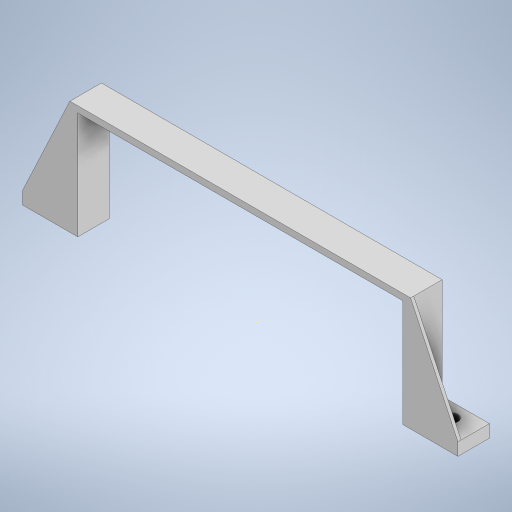
# Autodesk Inventor part: KVMMount
Saved by Autodesk Inventor 2023 (Build 270158000, 158)
## iProperties
Created: 2023-03-26
Part Number: KVMMount
Material: Generic
Document SubType Name: Modeling
Designer: lidang
Density: 1 g/cm^3
Appearance: Default
Author: lidang
Autodesk Inventor part; units mm, degrees
ref_plane "YZ Plane" through (0, 0, 0) normal (1, 0, 0) x (0, 1, 0)
ref_plane "XZ Plane" through (0, 0, 0) normal (0, 1, 0) x (-1, 0, 0)
ref_plane "XY Plane" through (0, 0, 0) normal (0, 0, 1) x (1, 0, 0)
sketch "Sketch1" plane through (0, 0, 0) normal (0, 0, 1) x (1, 0, 0)
  point P0 (0, 0)
sketch "Sketch2" plane through (0, 0, 0) normal (0, 0, 1) x (1, 0, 0)
  line L0 (-69, 0) -> (-69, 4)
  line L1 (-69, 4) -> (-54, 4)
  line L2 (-54, 4) -> (-54, 36)
  line L3 (-54, 36) -> (0, 36)
  line L4 (0, 36) -> (0, 34)
  line L5 (0, 34) -> (-51.5, 34)
  line L6 (-51.5, 34) -> (-51.5, 0)
  line L7 (-51.5, 0) -> (-69, 0)
  point P0 (0, 0)
  point P1 (-25.75, 34)
  point P2 (0, 35)
  dimension "d0" = 2
  dimension "d1" = 2.5
  dimension "d2" = 4
  dimension "d3" = 4
  dimension "d4" = 15
  dimension "d6" = 0
  dimension "d8" = 51.5
  dimension "d11" = 34
  constraints: 16 end point, 7 perpendicular, 2 midpoint, 1 vertical
  measures "d0" distance from line of point (-25.75, 34) L3
  measures "d1" distance between parallel lines of L6 L2
  measures "d2" distance from line of point (0, 0) L1
  measures "d3" distance between parallel lines of L1 L7
  measures "d4" distance between parallel lines of L0 L2
  measures "d6" horizontal distance of point (0, 0) point (0, 35)
  measures "d8" distance from line of point (0, 0) L6
  measures "d11" distance from line of point (0, 0) L5
extrude "Extrusion1" add sketch "Sketch2" along normal mid plane 10
mirror "Mirror1" about plane through (0, 34, 0) normal (1, 0, 0) of "Extrusion1"
sketch "Sketch3" plane through (0, 0, 5) normal (0, 0, 1) x (1, 0, 0)
  line L0 (-54, 36) -> (-54, 4) projected
  line L1 (-54, 36) -> (-54, 4)
  line L2 (-54, 4) -> (-69, 4) projected
  line L3 (-54, 4) -> (-69, 4)
  line L4 (-69, 4) -> (-54, 36)
  point P0 (0, 0)
  constraints: 6 end point, 1 collinear, 1 vertical
extrude "Extrusion2" add sketch "Sketch3" against normal blind 1
mirror "Mirror2" about plane through (0, 0, 0) normal (1, 0, 0) of "Extrusion2"
sketch "Sketch4" plane through (54, 4, -5) normal (0, 1, 0) x (1, 0, 0)
  circle A0 centre (7.5, -4.5) radius 1.9938
  line L0 (0, 0) -> (0, -9) projected
  line L1 (15, 0) -> (0, 0) projected
  point P0 (-54, -5)
  point P1 (0, -4.5)
  dimension "d14" = 7.5
  dimension "d15" = 4.5
  constraints: 1 centre point, 1 midpoint
  measures "d14" distance of point (0, -4.5) A0.centre
  measures "d15" distance from line of L1 A0.centre
extrude "Extrusion3" cut sketch "Sketch4" against normal blind 20
mirror "Mirror3" about plane through (0, 0, 0) normal (1, 0, 0) of "Extrusion3"
equation "\"d3\" = d2"
body "Solid1"
